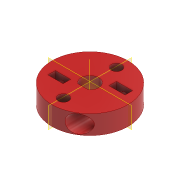
# Autodesk Inventor part: clamping hub .770 .25 D bore left
Saved by Autodesk Inventor 2020 (Build 240168000, 168)
## iProperties
Created: 2020-01-17
Part Number: clamping hub .770 .25 D bore left
Material: Generic
Document SubType Name: Modeling
Designer: ball
Density: 1 g/cm^3
Appearance: Default
Author: ball
Autodesk Inventor part; units mm, degrees
ref_plane "XZ Plane" through (0, 0, 0) normal (0, 1, 0) x (-1, 0, 0)
sketch "Sketch1" plane through (0, 0, 0) normal (0, 1, 0) x (-1, 0, 0)
  circle A0 centre (0, 0) radius 13.97
  dimension "d75" = 27.94
  constraints: 1 centre point
  measures "d75" diameter of A0
extrude "Extrusion1" add sketch "Sketch1" along normal blind 3.4925 and the other way blind 3.4925
ref_plane "Work Plane1" through (0, 0, 2.5) normal (0, 0, 1) x (1, 0, 0)
ref_plane "Work Plane2" through (0, 0, -2.5) normal (0, 0, 1) x (1, 0, 0)
sketch "Sketch2" plane through (0, 0, 0) normal (0, 0, 1) x (1, 0, 0)
  circle A0 centre (7.4168, 0) radius 1.7
  circle A1 centre (-7.4168, 0) radius 1.7
  point P0 (0, 0)
  dimension "d5" = 3.4
  dimension "d6" = 7.4168
  dimension "d7" = 3.4
  dimension "d8" = 7.4168
  constraints: 2 centre point
  measures "d5" diameter of A0
  measures "d6" distance of A0.centre point (0, 0)
  measures "d7" diameter of A1
  measures "d8" distance of A1.centre point (0, 0)
extrude "Screw hole 2" cut sketch "Sketch2" along normal blind 2.5 and the other way blind 6 contours A0
sketch "Sketch3" plane through (0, 0, 2.5) normal (0, 0, 1) x (1, 0, 0)
  circle A0 centre (7.4168, 0) radius 1.7 projected
  circle A1 centre (7.4168, 0) radius 3.25
  point P0 (0, 0)
  dimension "d19" = 6.5
  constraints: 1 centre point, 1 coincident
  measures "d19" diameter of A1
sketch "Sketch4" plane through (0, 0, -2.5) normal (0, 0, 1) x (1, 0, 0)
  circle A0 centre (7.4168, 0) radius 1.7 projected
  circle A1 centre (7.4168, 0) radius 3.45 construction
  line L0 (7.4168, -3.45) -> (4.429, -1.725)
  line L1 (4.429, -1.725) -> (4.429, 6.985)
  line L2 (10.4046, 6.985) -> (10.4046, -1.725)
  line L3 (10.4046, -1.725) -> (7.4168, -3.45)
  line L4 (10.4046, 6.985) -> (4.429, 6.985)
  point P0 (0, 0)
  dimension "d22" = 6.9
  constraints: 10 end point, 2 coincident, 1 vertical alignment, 8 other
sketch "Sketch5" plane through (0, 0, -2.5) normal (0, 0, 1) x (1, 0, 0)
  circle A0 centre (-7.422, 0) radius 3.25
  point P0 (0, 0)
  dimension "d25" = 6.5
  constraints: 1 centre point
  measures "d25" diameter of A0
extrude "Access Hole 1" cut sketch "Sketch5" against normal through all
extrude "Access Hole 2" cut sketch "Sketch3" along normal through all contours A0 | A1
extrude "Nut well 2" cut sketch "Sketch4" against normal blind 2.794 contours A0 | L0 L1 L4 L2 L3
sketch "Sketch7" plane through (0, 0, 2.5) normal (0, 0, 1) x (1, 0, 0)
  circle A0 centre (-7.422, 0) radius 3.25 construction
  circle A1 centre (-7.422, 0) radius 3.45 construction
  line L0 (-7.422, -3.25) -> (-10.2365, -1.625)
  line L1 (-10.2365, -1.625) -> (-10.2365, 5.3975)
  line L2 (-4.6074, 5.3975) -> (-4.6074, -1.625)
  line L3 (-4.6074, -1.625) -> (-7.422, -3.25)
  line L4 (16.6201, 5.3975) -> (-16.6201, 5.3975) projected
  line L5 (-10.2365, 5.3975) -> (-4.6074, 5.3975)
  point P0 (0, 0)
  dimension "d48" = 6.9
  constraints: 10 end point, 2 coincident, 2 point on line, 1 centre point, 1 vertical alignment, 7 other
  measures "d48" diameter of A1
extrude "Nut Well 1" cut sketch "Sketch7" along normal blind 2.794
sketch "Sketch8" plane through (0, 0, 0) normal (0, 0, 1) x (1, 0, 0)
  circle A0 centre (-7.422, 0) radius 3.25 projected
  circle A1 centre (-7.422, 0) radius 1.7
  point P0 (0, 0)
  dimension "d51" = 3.4
  constraints: 1 centre point, 1 coincident
  measures "d51" diameter of A1
extrude "Screw Hole 1" cut sketch "Sketch8" along normal blind 6 and the other way blind 2.5 contours A1
ref_plane "Work Plane3" through (0, 5.3975, 0) normal (0, 1, 0) x (1, 0, 0)
sketch "Sketch9" plane through (0, 5.3975, 0) normal (0, 1, 0) x (1, 0, 0)
  arc A0 (1.9431, -2.5908) -> (-1.9431, -2.5908) centre (0, 0) ccw
  line L0 (-1.9431, -2.5908) -> (1.9431, -2.5908)
  dimension "d56" = 6.477
  dimension "d57" = 2.5908
  constraints: 2 end point, 2 point on circle, 1 centre point, 1 coincident, 1 horizontal
  measures "d56" diameter of A0
  measures "d57" distance from line of L0 point (0, 0)
extrude "Center shaft" cut sketch "Sketch9" against normal through all
ref_plane "Work Plane4" through (0, 5.3975, 0) normal (0, 1, 0) x (1, 0, 0)
sketch "Sketch10" plane through (0, 5.3975, 0) normal (0, 1, 0) x (1, 0, 0)
  circle A0 centre (0, 9.779) radius 1.9304
  circle A1 centre (0, -9.779) radius 1.9304
  point P0 (0, 0)
  point P1 (0, -8.001)
  dimension "d60" = 3.8608
  dimension "d61" = 9.779
  dimension "d62" = 3.8608
  dimension "d63" = 9.779
  constraints: 2 centre point
  measures "d60" diameter of A0
  measures "d61" distance of A0.centre point (0, 0)
  measures "d62" diameter of A1
  measures "d63" distance of A1.centre point (0, 0)
extrude "Wheel holes" cut sketch "Sketch10" against normal through all
equation "\"d63\" = d61"
body "Solid1"
